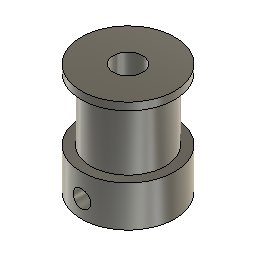
jakeRead_rotary-design-pattern (Autodesk Fusion 360 archive; units mm, degrees)
design "GT2 20T Pulley"
Autodesk Fusion 360 part; units mm, degrees
sketch "Sketch1" plane through (0, 0, 0) normal (0, 1, 0) x (1, 0, 0)
  line L0 (0, 0) -> (8, 0)
  line L1 (8, 0) -> (8, -7)
  line L2 (8, -7) -> (6.3662, -7)
  line L3 (6.3662, -7) -> (6.3662, -17.7)
  line L4 (6.3662, -17.7) -> (8, -17.7)
  line L5 (8, -17.7) -> (8, -19)
  line L6 (8, -19) -> (2.5, -19)
  line L7 (2.5, -19) -> (2.5, 0)
  circle A0 centre (0, -3) radius 1.5
  line L8 (0, 0) -> (0, -3) construction
  dimension "d1" = 2.5
  dimension "d2" = 8
  dimension "d3" = 7
  dimension "d4" = 6.3662
  dimension "d5" = 1.3
  dimension "d6" = 19
  dimension "d8" = 3
  dimension "d9" = 3
  constraint coincident L0.start L8.start
  constraint horizontal L0
  constraint perpendicular L0 L1
  constraint perpendicular L1 L2
  constraint perpendicular L2 L3
  constraint perpendicular L3 L4
  constraint perpendicular L4 L5
  constraint perpendicular L3 L6
  constraint coincident L0 L7.end
  constraint perpendicular L0 L7
  constraint coincident L1.end L5
  constraint coincident A0.centre L8.end
  constraint vertical L8
  measures "d1" distance of L0.start L7
  measures "d2" distance of L0.start L1
  measures "d3" distance of L0.end L1.end
  measures "d4" distance of L0.start L3
  measures "d5" distance of L4.end L5.end
  measures "d6" distance of L0.end L6
  measures "d8" diameter of A0
  measures "d9" distance of L0.start A0.centre
revolve "Revolve1" add sketch "Sketch1" angle 360 about axis through (0, 0, 1.75) along (0, 0, 1) contours L0 L1 L2 L3 L4 L5 L6 L7
extrude "Extrude1" cut sketch "Sketch1" against normal blind 17 contours A0
equation "d1 = ( 5 / 2 ) * 1 mm"
equation "d2 = ( 16 / 2 ) * 1 mm"
equation "d4 = ( 20 * 2 / PI ) * 1 mm / 2"

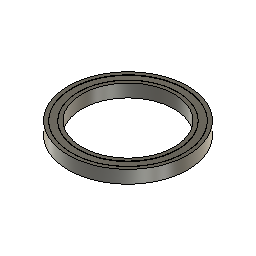
design "6808"
Autodesk Fusion 360 part; units mm, degrees
sketch "Sketch1" plane through (0, 0, 0) normal (0, 1, 0) x (1, 0, 0)
  line L0 (25, 0) -> (32.5, 0)
  line L1 (32.5, 0) -> (32.5, -7)
  line L2 (32.5, -7) -> (25, -7)
  line L3 (25, -7) -> (25, 0)
  line L4 (27, -7) -> (27, 0)
  line L5 (30.5, -7) -> (30.5, 0)
  line L6 (30.5, -6.75) -> (27, -6.75)
  line L7 (27, -0.25) -> (30.5, -0.25)
  dimension "d1" = 7
  dimension "d2" = 25
  dimension "d3" = 32.5
  dimension "d4" = 2
  dimension "d5" = 2
  dimension "d7" = 0.25
  dimension "d8" = 0.25
  constraint horizontal L0
  constraint vertical L1
  constraint horizontal L2
  constraint vertical L3
  constraint coincident origin L0
  constraint coincident L2 L4.start
  constraint coincident L0 L4.end
  constraint perpendicular L0 L4
  constraint coincident L2 L5.start
  constraint coincident L0 L5.end
  constraint perpendicular L0 L5
  constraint coincident L5 L6.start
  constraint coincident L4 L6.end
  constraint perpendicular L4 L6
  constraint coincident L4 L7.start
  constraint perpendicular L5 L7
  constraint coincident L5 L7.end
  measures "d1" distance of L0.end L1.end
  measures "d2" distance of origin L3
  measures "d3" distance of origin L1
  measures "d4" distance of L2.end L4
  measures "d5" distance of L1 L5
  measures "d7" distance of L5.end L7
  measures "d8" distance of L5.start L6.start
revolve "Revolve1" add sketch "Sketch1" angle 360 about axis through (0, 0, 1.75) along (0, 0, 1) contours L0 L2 L3 L4 | L0 L1 L2 L5 | L4 L5 L6 L7
equation "d2 = ( 50 / 2 ) * 1 mm"
equation "d3 = ( 65 / 2 ) * 1 mm"
equation "d8 = d7"

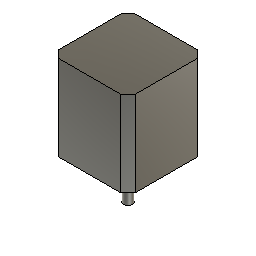
design "N17 48mm"
Autodesk Fusion 360 part; units mm, degrees
sketch "Sketch1" plane through (0, 0, 0) normal (0, 0, 1) x (1, 0, 0)
  line L0 (21.6, 21.6) -> (-21.6, 21.6)
  line L1 (-21.6, 21.6) -> (-21.6, -21.6)
  line L2 (-21.6, -21.6) -> (21.6, -21.6)
  line L3 (21.6, -21.6) -> (21.6, 21.6)
  line L4 (21.6, 21.6) -> (-21.6, -21.6) construction
  line L5 (-21.6, 21.6) -> (21.6, -21.6) construction
  circle A0 centre (0, 0) radius 11
  line L6 (-15.5, 15.5) -> (15.5, 15.5) construction
  line L7 (15.5, 15.5) -> (15.5, -15.5) construction
  line L8 (15.5, -15.5) -> (-15.5, -15.5) construction
  line L9 (-15.5, -15.5) -> (-15.5, 15.5) construction
  circle A1 centre (-15.5, 15.5) radius 1.5
  circle A2 centre (-15.5, -15.5) radius 1.5
  circle A3 centre (15.5, -15.5) radius 1.5
  circle A4 centre (15.5, 15.5) radius 1.5
  circle A5 centre (0, 0) radius 2.5
  dimension "d1" = 43.2
  dimension "d2" = 22
  dimension "d3" = 31
  dimension "d4" = 3
  dimension "d5" = 5
  constraint perpendicular L0 L1
  constraint parallel L0 L2
  constraint parallel L1 L3
  constraint horizontal L0
  constraint coincident L4 A0.centre
  constraint coincident L5 A0.centre
  constraint coincident A0.centre A5.centre
  constraint equal L0 L1
  constraint horizontal L6
  constraint vertical L7
  constraint horizontal L8
  constraint vertical L9
  constraint coincident L5 L7.end
  constraint coincident L5 L6.start
  constraint coincident L4 L6.end
  constraint coincident L6.start L9.end
  constraint coincident L8.end L9.start
  constraint coincident L7.end L8.start
  constraint coincident L6.end L7.start
  constraint equal A1 A4
  constraint equal A1 A2
  constraint equal A1 A3
  constraint concentric A0 A5
  measures "d1" distance of L0.start L0.end
  measures "d2" diameter of A0
  measures "d3" distance of L6.start L6.end
  measures "d4" diameter of A1
  measures "d5" diameter of A5
extrude "Extrude1" add sketch "Sketch1" along normal blind 48 contours L0 L1 L2 L3 | A0 | A1 | A2 | A3 | A4 | A5
extrude "Extrude2" cut sketch "Sketch1" along normal blind 5 contours A1 | A2 | A3 | A4
extrude "Extrude3" add sketch "Sketch1" against normal blind 2 contours A0 | A5
extrude "Extrude4" add sketch "Sketch1" against normal blind 24 contours A5
chamfer "Chamfer1" distance 4 angle 45 4 edges at (-21.6, -21.6, 24) (-21.6, 21.6, 24) (21.6, -21.6, 24) (21.6, 21.6, 24)
